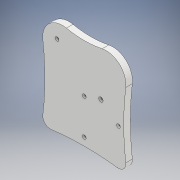
# Autodesk Inventor part: Chwytaka3_o
Saved by Autodesk Inventor 2017 (Build 210142000, 142)
## iProperties
Created: 2014-11-16
Part Number: Chwytaka3_o
Material: SolidWorks Materials|ABS
Document SubType Name: Modeling
Designer: Maciej
Density: 1.02 g/cm^3
Appearance: 255,255,255
Sending System: SolidWorks 2013
Last Author: Raymond Ma
Last Saved: 2015-02-18
Author: Maciej
Autodesk Inventor part; units mm, degrees
ref_plane "YZ Plane" through (0, 0, 0) normal (1, 0, 0) x (0, 1, 0)
ref_plane "XZ Plane" through (0, 0, 0) normal (0, 1, 0) x (-1, 0, 0)
ref_plane "XY Plane" through (0, 0, 0) normal (0, 0, 1) x (1, 0, 0)
sketch "Szkic2" plane through (0, 0, 0) normal (0, 1, 0) x (-1, 0, 0)
  arc A0 (47.3256, 42.282) -> (47.3256, -32.282) centre (345, 5) ccw projected
  arc A1 (47.3256, 42.282) -> (20.4082, 67.1046) centre (25, 45.0782) ccw projected
  arc A2 (47.3256, 42.282) -> (20.4082, 67.1046) centre (25, 45.0782) ccw
  arc A3 (47.3256, 42.282) -> (47.3256, -32.282) centre (347.6289, 5) ccw
  arc A4 (-20.4082, 67.1046) -> (20.4082, 67.1046) centre (0, 165) ccw projected
  arc A5 (-20.4082, 67.1046) -> (20.4082, 67.1046) centre (0, 165) ccw
  arc A6 (-20.4082, 67.1046) -> (-47.3256, 42.282) centre (-25, 45.0782) ccw projected
  arc A7 (-20.4082, 67.1046) -> (-20.4082, 67.1046) centre (-25, 45.0782) ccw
  arc A8 (-47.3256, -32.282) -> (-47.3256, 42.282) centre (-345, 5) ccw projected
  arc A9 (-20.4082, 67.1046) -> (-47.3256, 42.282) centre (-25, 45.0782) ccw
  arc A10 (-47.3256, -32.282) -> (-47.3256, 42.282) centre (-345, 5) ccw
  arc A11 (37.8287, -41.7716) -> (-37.8287, -41.7716) centre (0, -341.9445) ccw projected
  arc A12 (-47.3256, -32.282) -> (-37.8287, -41.7716) centre (-38.8915, -33.3383) ccw
  arc A13 (-47.3256, -32.282) -> (-37.8287, -41.7716) centre (-38.8915, -33.3383) ccw projected
  arc A14 (37.8287, -41.7716) -> (-37.8287, -41.7716) centre (0, -341.9445) ccw
  arc A15 (37.8287, -41.7716) -> (47.3256, -32.282) centre (38.8915, -33.3383) ccw projected
  arc A16 (38.2038, -38.7952) -> (44.3488, -32.6548) centre (38.8915, -33.3383) ccw projected
  arc A17 (38.2038, -38.7952) -> (44.3488, -32.6548) centre (38.8915, -33.3383) ccw
  arc A18 (44.3488, 42.6548) -> (44.3488, -32.6548) centre (345, 5) ccw projected
  arc A19 (44.3488, -32.6548) -> (44.3488, -32.6548) centre (345, 5) ccw
  arc A20 (44.3488, 42.6548) -> (21.0204, 64.1678) centre (25, 45.0782) ccw projected
  arc A21 (-21.0204, 64.1678) -> (21.0204, 64.1678) centre (0, 165) ccw projected
  arc A22 (21.0204, 64.1678) -> (21.0204, 64.1678) centre (0, 165) ccw
  arc A23 (-21.0204, 64.1678) -> (-44.3488, 42.6548) centre (-25, 45.0782) ccw projected
  arc A24 (-21.0204, 64.1678) -> (-44.3488, 42.6548) centre (-25, 45.0782) ccw
  arc A25 (-44.3488, -32.6548) -> (-38.2038, -38.7952) centre (-38.8915, -33.3383) ccw projected
  arc A26 (-30.075, -37.8811) -> (-38.2038, -38.7952) centre (0, -341.9445) ccw projected
  arc A27 (38.2038, -38.7952) -> (27.846, -37.6689) centre (0, -341.9445) ccw projected
  arc A28 (27.846, -37.6689) -> (-30.075, -37.8811) centre (0, -341.9445) ccw
  circle A29 centre (0, 10) radius 2.1526 projected
  circle A30 centre (0, 10) radius 2.1526
  circle A31 centre (0, -30.3974) radius 2.1526 projected
  circle A32 centre (0, -30.3974) radius 2.1526
  circle A33 centre (-39, 0) radius 2.1526 projected
  circle A34 centre (-39, 0) radius 2.1526
  circle A35 centre (31.0104, 51.0886) radius 2.1526 projected
  circle A36 centre (31.0104, 51.0886) radius 2.1526
  arc A37 (-42.0195, 1.5629) -> (-44.3488, 42.6548) centre (-345, 5) ccw projected
  arc A38 (-44.3488, 42.6548) -> (-44.3488, 42.6548) centre (-345, 5) ccw
  arc A39 (-42.0195, 1.5629) -> (-42.0689, -1.4634) centre (-39, 0) ccw projected
  arc A40 (-42.0195, 1.5629) -> (-42.0195, 1.5629) centre (-39, 0) ccw
  arc A41 (-44.3488, -32.6548) -> (-42.0689, -1.4634) centre (-345, 5) ccw projected
  arc A42 (-42.0689, -1.4634) -> (-42.0689, -1.4634) centre (-345, 5) ccw
  line L0 (5.5773, 31.6985) -> (5.5773, 17.4485)
  line L1 (5.5773, 31.6985) -> (5.5773, 45.9485)
  line L2 (5.5773, 17.4485) -> (5.5773, 45.9485)
  line L3 (5.5773, 45.9485) -> (5.5773, 17.4485)
  line L4 (5.5773, 23.6985) -> (-6.4227, 23.6985)
  line L5 (-6.4227, 39.6985) -> (5.5773, 39.6985)
  line L6 (5.5773, 39.6985) -> (5.5773, 23.6985)
  line L7 (5.5773, 45.9485) -> (-6.4227, 45.9485)
  line L8 (-6.4227, 45.9485) -> (-6.4227, 39.6985)
  line L9 (-6.4227, 39.6985) -> (5.5773, 39.6985)
  line L10 (5.5773, 39.6985) -> (5.5773, 45.9485)
  line L11 (5.5773, 17.4485) -> (-6.4227, 17.4485)
  line L12 (-6.4227, 17.4485) -> (-6.4227, 23.6985)
  line L13 (-6.4227, 23.6985) -> (5.5773, 23.6985)
  line L14 (5.5773, 23.6985) -> (5.5773, 17.4485)
  line L15 (-6.4227, 23.6985) -> (5.5773, 23.6985)
  line L16 (5.5773, 23.6985) -> (5.5773, 39.6985)
  line L17 (5.5773, 39.6985) -> (-6.4227, 39.6985)
  line L18 (-6.4227, 39.6985) -> (-6.4227, 23.6985)
  line L19 (35.2412, 7.5499) -> (35.2412, -26.4501)
  line L20 (35.2412, -26.4501) -> (33.7412, -26.4501)
  line L21 (33.7412, -26.4501) -> (33.7412, 7.5499)
  line L22 (33.7412, 7.5499) -> (33.7412, -26.4501)
  line L23 (19.4912, -26.4501) -> (33.7412, -26.4501)
  line L24 (5.2412, -26.4501) -> (5.2412, 7.5499)
  line L25 (5.2412, -26.4501) -> (5.2412, 7.5499)
  line L26 (3.7412, 7.5499) -> (3.7412, -26.4501)
  line L27 (19.4912, -26.4501) -> (5.2412, -26.4501)
  line L28 (28.0412, 9.0499) -> (28.0412, 7.5499)
  line L29 (5.2412, 7.5499) -> (33.7412, 7.5499)
  line L30 (33.7412, 7.5499) -> (35.2412, 7.5499)
  line L31 (28.0412, 7.5499) -> (35.2412, 7.5499)
  line L32 (35.2412, 9.0499) -> (28.0412, 9.0499)
  line L33 (35.2412, 7.5499) -> (35.2412, 9.0499)
  line L34 (5.2412, 7.5499) -> (3.7412, 7.5499)
  line L35 (10.9412, 7.5499) -> (3.7412, 7.5499)
  line L36 (3.7412, 9.0499) -> (10.9412, 9.0499)
  line L37 (3.7412, 7.5499) -> (3.7412, 9.0499)
  line L38 (10.9412, 9.0499) -> (10.9412, 7.5499)
  line L39 (33.7412, -26.4501) -> (5.2412, -26.4501)
  line L40 (3.7412, -26.4501) -> (5.2412, -26.4501)
  line L41 (5.2412, -26.4501) -> (33.7412, -26.4501)
  line L42 (27.4912, -26.4501) -> (27.4912, -38.4501)
  line L43 (11.4912, -38.4501) -> (11.4912, -26.4501)
  line L44 (11.4912, -26.4501) -> (27.4912, -26.4501)
  line L45 (5.2412, -26.4501) -> (5.2412, -38.4501)
  line L46 (5.2412, -38.4501) -> (11.4912, -38.4501)
  line L47 (11.4912, -38.4501) -> (11.4912, -26.4501)
  line L48 (11.4912, -26.4501) -> (5.2412, -26.4501)
  line L49 (33.7412, -26.4501) -> (33.7412, -38.4501)
  line L50 (33.7412, -38.4501) -> (27.4912, -38.4501)
  line L51 (27.4912, -38.4501) -> (27.4912, -26.4501)
  line L52 (27.4912, -26.4501) -> (33.7412, -26.4501)
  line L53 (27.4912, -38.4501) -> (27.4912, -26.4501)
  line L54 (27.4912, -26.4501) -> (11.4912, -26.4501)
  line L55 (11.4912, -26.4501) -> (11.4912, -38.4501)
  line L56 (11.4912, -38.4501) -> (27.4912, -38.4501)
  line L57 (-27.4912, -26.4501) -> (-33.7412, -26.4501)
  line L58 (-33.7412, 7.5499) -> (-35.2412, 7.5499)
  line L59 (-5.2412, 7.5499) -> (-3.7412, 7.5499)
  line L60 (-11.4912, -38.4501) -> (-11.4912, -26.4501)
  line L61 (-11.4912, -38.4501) -> (-11.4912, -26.4501)
  line L62 (-11.4912, -26.4501) -> (-11.4912, -38.4501)
  line L63 (5.5773, 47.4485) -> (5.5773, 45.9485)
  line L64 (39.5773, 45.9485) -> (39.5773, 47.4485)
  line L65 (39.5773, 15.9485) -> (39.5773, 17.4485)
  line L66 (5.5773, 45.9485) -> (5.5773, 17.4485)
  line L67 (5.5773, 47.4485) -> (39.5773, 47.4485)
  line L68 (39.5773, 47.4485) -> (39.5773, 45.9485)
  line L69 (39.5773, 45.9485) -> (5.5773, 45.9485)
  line L70 (5.5773, 45.9485) -> (5.5773, 47.4485)
  line L71 (39.5773, 15.9485) -> (5.5773, 15.9485)
  line L72 (5.5773, 15.9485) -> (5.5773, 17.4485)
  line L73 (5.5773, 17.4485) -> (39.5773, 17.4485)
  line L74 (39.5773, 17.4485) -> (39.5773, 15.9485)
  line L75 (39.5773, 47.4485) -> (41.0773, 47.4485)
  line L76 (41.0773, 47.4485) -> (41.0773, 40.2485)
  line L77 (41.0773, 40.2485) -> (39.5773, 40.2485)
  line L78 (39.5773, 40.2485) -> (39.5773, 47.4485)
  line L79 (39.5773, 15.9485) -> (41.0773, 15.9485)
  line L80 (41.0773, 15.9485) -> (41.0773, 23.1485)
  line L81 (41.0773, 23.1485) -> (39.5773, 23.1485)
  line L82 (39.5773, 23.1485) -> (39.5773, 15.9485)
  line L83 (39.5773, 45.9485) -> (5.5773, 45.9485)
  line L84 (5.5773, 45.9485) -> (5.5773, 17.4485)
  line L85 (5.5773, 17.4485) -> (39.5773, 17.4485)
  line L86 (39.5773, 17.4485) -> (39.5773, 45.9485)
  line L87 (-5.2412, -26.4501) -> (-3.7412, -26.4501)
  line L88 (-3.7412, -26.4501) -> (-3.7412, 7.5499)
  line L89 (-3.7412, 7.5499) -> (-5.2412, 7.5499)
  line L90 (-5.2412, 7.5499) -> (-5.2412, -26.4501)
  line L91 (-33.7412, -26.4501) -> (-35.2412, -26.4501)
  line L92 (-35.2412, -26.4501) -> (-35.2412, 7.5499)
  line L93 (-35.2412, 7.5499) -> (-33.7412, 7.5499)
  line L94 (-33.7412, 7.5499) -> (-33.7412, -26.4501)
  line L95 (-3.7412, 7.5499) -> (-10.9412, 7.5499)
  line L96 (-10.9412, 7.5499) -> (-10.9412, 9.0499)
  line L97 (-10.9412, 9.0499) -> (-3.7412, 9.0499)
  line L98 (-3.7412, 9.0499) -> (-3.7412, 7.5499)
  line L99 (-35.2412, 7.5499) -> (-28.0412, 7.5499)
  line L100 (-28.0412, 7.5499) -> (-28.0412, 9.0499)
  line L101 (-28.0412, 9.0499) -> (-35.2412, 9.0499)
  line L102 (-35.2412, 9.0499) -> (-35.2412, 7.5499)
  line L103 (-33.7412, -26.4501) -> (-33.7412, 7.5499)
  line L104 (-5.2412, 7.5499) -> (-5.2412, -26.4501)
  line L105 (-27.4912, -26.4501) -> (-27.4912, -38.4501)
  line L106 (-27.4912, -38.4501) -> (-11.4912, -38.4501)
  line L107 (-11.4912, -38.4501) -> (-11.4912, -26.4501)
  line L108 (-11.4912, -38.4501) -> (-5.2412, -38.4501)
  line L109 (-5.2412, -38.4501) -> (-5.2412, -26.4501)
  line L110 (-5.2412, -26.4501) -> (-11.4912, -26.4501)
  line L111 (-11.4912, -26.4501) -> (-11.4912, -38.4501)
  line L112 (-33.7412, -26.4501) -> (-27.4912, -26.4501)
  line L113 (-27.4912, -26.4501) -> (-27.4912, -38.4501)
  line L114 (-27.4912, -38.4501) -> (-33.7412, -38.4501)
  line L115 (-33.7412, -38.4501) -> (-33.7412, -26.4501)
  line L116 (-33.7412, 7.5499) -> (-5.2412, 7.5499)
  line L117 (-5.2412, 7.5499) -> (-5.2412, -26.4501)
  line L118 (-5.2412, -26.4501) -> (-33.7412, -26.4501)
  line L119 (-33.7412, -26.4501) -> (-33.7412, 7.5499)
  point P0 (6, 11.2)
  point P1 (26, 46.0782)
  point P2 (26, 46.0782)
  point P3 (26, 46.0782)
  point P4 (26, 46.0782)
  point P5 (-6.4227, 23.6985)
  point P6 (5.6006, -7.3555)
  point P7 (4.6006, -6.3555)
  point P8 (4.6006, -6.3555)
  point P9 (4.6006, -6.3555)
  point P10 (4.6006, -6.3555)
  point P11 (26.9803, -38.7782)
  point P12 (-26.9803, -38.7782)
  point P13 (-5.6006, -7.3555)
  point P14 (-4.6006, -6.3555)
  point P15 (-4.6006, -6.3555)
  point P16 (-4.6006, -6.3555)
  point P17 (-4.6006, -6.3555)
  dimension "d43" = 14.25
  dimension "d44" = 14.25
  dimension "d118" = 14.25
  dimension "d119" = 14.25
  dimension "d122" = 34
  dimension "d123" = 1.5
  dimension "d124" = 7.2
  dimension "d125" = 1.5
  dimension "d126" = 34
  dimension "d127" = 1.5
  dimension "d129" = 7.2
  dimension "d130" = 28.5
  dimension "d142" = 1.5
  dimension "d143" = 7.2
  dimension "d144" = 7.2
  dimension "d145" = 7.2
  dimension "d146" = 7.2
  constraints: 240 end point, 51 parallel, 23 perpendicular, 20 point on circle, 16 horizontal, 14 centre point, 4 coincident, 3 concentric, 3 point on line, 1 tangent, 25 other
  measures "d43" distance of L0.start L0.end
  measures "d44" distance of L0.start L1.end
  measures "d118" distance of L23.start L20.end
  measures "d119" distance of L23.start L39.end
  measures "d122" distance of L30.end L19.end
  measures "d123" distance of L28.start L28.end
  measures "d124" distance of L32.start L28.start
  measures "d125" distance of L19.end L20.end
  measures "d126" distance of L26.end L26.start
  measures "d127" distance of L26.end L39.end
  measures "d129" distance of L36.start L36.end
  measures "d130" distance of L29.start L30.start
  measures "d142" distance of L76.end L77.end
  measures "d143" distance of L79.end L80.end
  measures "d144" distance of L75.end L76.end
  measures "d145" distance of L96.end L97.end
  measures "d146" distance of L101.end L100.end
extrude "Wyciągnięcie proste9" add sketch "Szkic2" along normal blind 5.8 contours L5 L1 L0 L4 L18 A7 | A7 L18 L5
extrude "Wyciągnięcie proste11" add sketch "Szkic2" along normal blind 5.8 contours L7 L1 L5 A7 | A7 L5 L8 L7
extrude "Wyciągnięcie proste12" add sketch "Szkic2" along normal blind 5.8 contours L4 L0 L11 L12
extrude "Wyciągnięcie proste20" add sketch "Szkic2" along normal blind 12 contours L21 L30 L19 L20 | L63 L67 L64 L69 | L29 L28 L32 L33 L30 | L64 L75 L76 L77 L78 | L91 L92 L58 L94 | L29 L34 L37 L36 L38 | L81 L80 L79 L65 L82 | L58 L102 L101 L100 L99 | L40 L26 L34 L24 | L73 L65 L71 L72 | L90 L59 L88 L87 | L96 L97 L98 L59 L95
extrude "Wyciągnięcie proste21" add sketch "Szkic2" along normal blind 5.8 contours L42 L56 L43 A28 | A28 L43 L27 L23 L42 | L105 L118 L60 A28 | A28 L60 L106 L105
extrude "Wyciągnięcie proste22" add sketch "Szkic2" along normal blind 5.8 contours L49 L50 L42 A28 A27 | A27 A28 L42 L23 L49 | L23 L27 L24 L29 L21 | L69 L78 L86 L82 L73 L0 L1 | L115 L57 L105 A28 A26 | A26 A28 L105 L114 L115 | L43 L46 L45 A28 | A28 L45 L27 L43 | L94 L99 L116 L95 L90 L110 L118 L57 | L109 L108 L60 A28 | A28 L60 L110 L109
extrude "Wyciągnięcie proste24" add sketch "Szkic2" along normal blind 1.5 contours A18 A16 A27 L49 L20 L19 L33 L32 L28 L29 L38 L36 L37 L26 L40 L45 A28 L109 L87 L88 L98 L97 L96 L116 L100 L101 L102 L92 L91 L115 A26 A25 A38 A40 A37 A7 L18 L12 L11 L72 L71 L79 L80 L81 L86 L77 L76 L75 L67 L63 L7 A21 A20 | A7 L7 L8 L18 A37 A23 A21 | A39 A38 | A38 A40
extrude "Wyciągnięcie proste25" add sketch "Szkic2" against normal blind 1 contours A0 A15 A19 A18 A1 | A19 A20 A22 A1 | A15 A11 A12 A38 A25 A26 L115 L114 L106 L108 L109 A28 L45 L46 L56 L50 L49 A27 A16 A19 | A22 A21 A7 A4 A1 | A18 A16 A27 L49 L20 L19 L33 L32 L28 L29 L38 L36 L37 L26 L40 L45 A28 L109 L87 L88 L98 L97 L96 L116 L100 L101 L102 L92 L91 L115 A26 A25 A38 A40 A37 A7 L18 L12 L11 L72 L71 L79 L80 L81 L86 L77 L76 L75 L67 L63 L7 A21 A20 | A7 A21 A22 A6 | A7 L7 L8 L18 A37 A23 A21 | A12 A8 A7 A37 A39 A38 | L49 L50 L42 A28 A27 | A27 A28 L42 L23 L49 | A22 A23 A38 A6 | L7 L1 L5 A7 | A7 L5 L8 L7 | L21 L30 L19 L20 | L23 L27 L24 L29 L21 | A38 A37 A7 A6 | L69 L78 L86 L82 L73 L0 L1 | L63 L67 L64 L69 | A39 A38 | A38 A40 | L42 L56 L43 A28 | A28 L43 L27 L23 L42 | L29 L28 L32 L33 L30 | L5 L1 L0 L4 L18 A7 | A7 L18 L5 | L64 L75 L76 L77 L78 | L115 L57 L105 A28 A26 | A26 A28 L105 L114 L115 | L43 L46 L45 A28 | A28 L45 L27 L43 | L94 L99 L116 L95 L90 L110 L118 L57 | L91 L92 L58 L94 | L29 L34 L37 L36 L38 | L4 L0 L11 L12 | L81 L80 L79 L65 L82 | L105 L118 L60 A28 | A28 L60 L106 L105 | L58 L102 L101 L100 L99 | L109 L108 L60 A28 | A28 L60 L110 L109 | L40 L26 L34 L24 | L73 L65 L71 L72 | L90 L59 L88 L87 | L96 L97 L98 L59 L95
sketch "Szkic5" plane through (-41.0773, 12, 15.9485) normal (-1, 0, 0) x (0, 0, 1)
  line L0 (0, 0) -> (7.2, 0) projected
  line L1 (1.5, -6.2) -> (1.5, 0) projected
  line L2 (1.5, -2.95) -> (4.75, -2.95)
  line L3 (4.75, -2.95) -> (4.75, 0)
  circle A0 centre (4.75, -2.95) radius 1
  point P0 (-15.9485, -12)
  dimension "d190" = 3.25
  dimension "d191" = 2
  constraints: 4 end point, 2 point on line, 1 centre point, 1 coincident, 1 perpendicular
  measures "d190" distance of L2.start L2.end
  measures "d191" diameter of A0
extrude "Wyciągnięcie proste26" cut sketch "Szkic5" against normal blind 2 contours A0 L2 L3 | L3 L2 A0
sketch "Szkic6" plane through (-41.0773, 12, 40.2485) normal (-1, 0, 0) x (0, 0, 1)
  line L0 (5.7, 0) -> (0, 0) projected
  line L1 (5.7, -6.2) -> (5.7, 0) projected
  line L2 (5.7, -2.95) -> (2.45, -2.95)
  line L3 (2.45, -2.95) -> (2.45, 0)
  circle A0 centre (2.45, -2.95) radius 1
  point P0 (-40.2485, -12)
  dimension "d195" = 3.25
  dimension "d196" = 2
  constraints: 4 end point, 2 point on line, 1 centre point, 1 coincident, 1 horizontal, 1 vertical
  measures "d195" distance of L2.start L2.end
  measures "d196" diameter of A0
extrude "Wyciągnięcie proste27" cut sketch "Szkic6" against normal blind 2 contours A0 L2 L3 | L3 L2 A0
sketch "Szkic7" plane through (28.0412, 12, 9.0499) normal (0, 0, 1) x (1, 0, 0)
  line L0 (5.7, 0) -> (5.7, -6.2) projected
  line L1 (5.7, -3.0106) -> (2.45, -3.0106)
  circle A0 centre (2.45, -3.0106) radius 1
  point P0 (-28.0412, -12)
  dimension "d200" = 3.25
  dimension "d201" = 2
  constraints: 2 end point, 1 centre point, 1 coincident, 1 horizontal, 1 point on line
  measures "d200" distance of L1.start L1.end
  measures "d201" diameter of A0
extrude "Wyciągnięcie proste28" cut sketch "Szkic7" against normal blind 2
sketch "Szkic8" plane through (3.7412, 12, 9.0499) normal (0, 0, 1) x (1, 0, 0)
  line L0 (7.2, 0) -> (1.5, 0) projected
  line L1 (1.5, -6.2) -> (1.5, 0) projected
  line L2 (1.5, -2.95) -> (4.75, -2.95)
  circle A0 centre (4.75, -2.95) radius 1
  point P0 (-3.7412, -12)
  dimension "d205" = 3.25
  dimension "d206" = 2
  constraints: 2 end point, 1 centre point, 1 coincident, 1 horizontal, 1 point on line
  measures "d205" distance of L2.start L2.end
  measures "d206" diameter of A0
extrude "Wyciągnięcie proste29" cut sketch "Szkic8" against normal blind 2
sketch "Szkic9" plane through (-10.9412, 12, 9.0499) normal (0, 0, 1) x (1, 0, 0)
  line L0 (5.7, 0) -> (5.7, -6.2) projected
  line L1 (5.7, 0) -> (5.7, -2.95)
  line L2 (5.7, -2.95) -> (2.45, -2.95)
  circle A0 centre (2.45, -2.95) radius 1
  point P0 (10.9412, -12)
  dimension "d209" = 2.95
  dimension "d210" = 3.25
  dimension "d211" = 2
  constraints: 4 end point, 1 centre point, 1 coincident, 1 horizontal, 1 point on line
  measures "d209" distance of L0.start L1.end
  measures "d210" distance of L1.end L2.end
  measures "d211" diameter of A0
extrude "Wyciągnięcie proste30" cut sketch "Szkic9" against normal blind 2
sketch "Szkic10" plane through (-35.2412, 12, 9.0499) normal (0, 0, 1) x (1, 0, 0)
  line L0 (7.2, 0) -> (1.5, 0) projected
  line L1 (1.5, -6.2) -> (1.5, 0) projected
  line L2 (1.5, -2.95) -> (4.75, -2.95)
  circle A0 centre (4.75, -2.95) radius 1
  point P0 (35.2412, -12)
  dimension "d215" = 3.25
  dimension "d216" = 2
  constraints: 2 end point, 1 centre point, 1 coincident, 1 horizontal, 1 point on line
  measures "d215" distance of L2.start L2.end
  measures "d216" diameter of A0
extrude "Wyciągnięcie proste31" cut sketch "Szkic10" against normal blind 2
extrude "Wyciągnięcie proste34" add sketch "Szkic2" along normal blind 6.5 contours A0 A15 A19 A18 A1 | A19 A20 A22 A1 | A15 A11 A12 A38 A25 A26 L115 L114 L106 L108 L109 A28 L45 L46 L56 L50 L49 A27 A16 A19 | A22 A21 A7 A4 A1 | A7 A21 A22 A6 | A12 A8 A7 A37 A39 A38 | A22 A23 A38 A6 | A38 A37 A7 A6
sketch "Szkic16" plane through (33.7412, 5.8, -38.4501) normal (0, 0, -1) x (-1, 0, 0)
  line L0 (0, 0) -> (28.5, 0) projected
  line L1 (22.8, 0) -> (28.5, 0) projected
  arc A0 (2.8005, 0) -> (25.7005, 0) centre (14.2505, 13.0945) ccw
  line L2 (12.7208, -4.3) -> (54.7616, -4.3) projected
  point P0 (33.7412, -5.8)
  dimension "d231" = 22.9
  constraints: 2 point on circle, 2 point on line, 1 centre point, 1 tangent
  measures "d231" distance of A0.start A0.end
sketch "Szkic17" plane through (-5.2412, 5.8, -38.4501) normal (0, 0, -1) x (-1, 0, 0)
  line L0 (0, 0) -> (28.5, 0) projected
  arc A0 (2.7997, 0) -> (25.6997, 0) centre (14.2497, 13.0945) ccw
  line L1 (35.8361, -4.3) -> (0.3361, -4.3) projected
  point P0 (-5.2412, -5.8)
  dimension "d232" = 22.9
  constraints: 2 point on circle, 2 point on line, 1 centre point, 1 tangent
  measures "d232" distance of A0.start A0.end
extrude "Wyciągnięcie proste35" cut sketch "Szkic16" against normal blind 12
extrude "Wyciągnięcie proste36" cut sketch "Szkic17" against normal blind 12
sketch "Szkic20" plane through (6.4227, 5.8, 45.9485) normal (1, 0, 0) x (0, 0, -1)
  line L0 (0, 0) -> (5.7, 0) projected
  line L1 (22.8, 0) -> (28.5, 0) projected
  arc A0 (2.7998, 0) -> (25.6998, 0) centre (14.2498, 13.0945) ccw
  line L2 (3.2936, -4.3) -> (44.3856, -4.3) projected
  point P0 (45.9485, -5.8)
  dimension "d239" = 22.9
  constraints: 2 point on circle, 2 point on line, 1 centre point, 1 tangent
  measures "d239" distance of A0.start A0.end
extrude "Wyciągnięcie proste37" cut sketch "Szkic20" against normal blind 12 fills toward (14.2498, -4.25) open curves A0
fillet "Zaokrąglenie3" radius 2 6 edges at (30.9407, 5.8, -32.4501) (8.0407, 5.8, -32.4501) (-8.0408, 5.8, -32.4501) (-30.9408, 5.8, -32.4501) (0.4227, 5.8, 43.1487) (0.4227, 5.8, 20.2487)
sketch "Szkic21" plane through (0, 1.5, 0) normal (0, 1, 0) x (1, 0, 0)
  circle A0 centre (0, -10) radius 2.1526 projected
  circle A1 centre (19, -16.245) radius 2.5
  point P0 (0, 0)
  dimension "d246" = 5
  constraints: 1 centre point
  measures "d246" diameter of A1
hole "Otwór6" at (19, 1.5, 16.245) direction (0, -1, 0) diameter 5 depth 8
